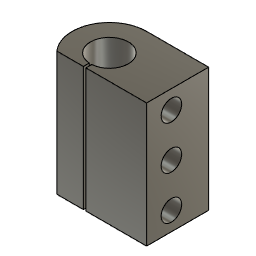
X-Idler (Autodesk Fusion 360 design; units mm, degrees)
Autodesk Fusion 360 part; units mm, degrees
note: some values were not read from the file. Set by a fixed rule: which sketch regions a step uses.
sketch "Skizze1" plane through (0, 0, 0) normal (0, 0, 1) x (1, 0, 0)
  circle A0 centre (0, 0) radius 7.65
  line L0 (15, -10) -> (-15, -10)
  line L1 (-15, -10) -> (-15, 15)
  line L2 (-15, 15) -> (15, 15)
  line L3 (15, 15) -> (15, -10)
  line L4 (0, 0) -> (0, -10)
  line L5 (0, -10) -> (-0.5, -10)
  line L6 (-0.5, -10) -> (0.5, -10)
  line L7 (0.5, -10) -> (0.5, -7.3)
  line L8 (0.5, -7.3) -> (-0.5, -7.3)
  line L9 (-0.5, -7.3) -> (-0.5, -10)
  circle A1 centre (0, 0) radius 15
  dimension "d1" = 15.3
  dimension "d4" = 15
  dimension "d5" = 10
  dimension "d6" = 15
  dimension "d7" = 25
  constraint coincident A0.centre L4.start
  constraint horizontal L0
  constraint vertical L1
  constraint horizontal L2
  constraint vertical L3
  constraint coincident L0 L4.end
  constraint perpendicular L0 L4
  constraint coincident L0 L5.end
  constraint horizontal L6
  constraint vertical L7
  constraint horizontal L8
  constraint vertical L9
  constraint concentric A0 A1
  constraint tangent L1 A1
  measures "d1" diameter of A0
  measures "d4" distance of A0.centre L3
  measures "d5" distance of A0.centre L0
  measures "d6" distance of A0.centre L1
  measures "d7" distance of L0.start L2.end
extrude "Extrusion1" add sketch "Skizze1" along normal blind 50 contours A0 L0 L7 L9 A1 | L0 L3 A1 | L2 L3 A1
sketch "Skizze2" plane through (15, 0, 0) normal (1, 0, 0) x (0, 1, 0)
  line L0 (-10, 0) -> (15, 0)
  line L1 (15, 0) -> (15, 50)
  line L2 (15, 50) -> (-10, 50)
  line L3 (-10, 50) -> (-10, 0)
  line L4 (-10, 25) -> (15, 25)
  circle A0 centre (0, 25) radius 4.15
  line L5 (0, 25) -> (0, 42.5)
  line L6 (0, 25) -> (0, 7.5)
  circle A1 centre (0, 42.5) radius 4.15
  circle A2 centre (0, 7.5) radius 4.15
  dimension "d10" = 8.3
  dimension "d11" = 10
  dimension "d22" = 17.5
  dimension "d23" = 8.3
  dimension "d24" = 8.3
  dimension "d25" = 17.5
  constraint midpoint L3 L4.start
  constraint midpoint L1 L4.end
  constraint coincident L4 A0.centre
  constraint coincident A0.centre L5.start
  constraint perpendicular L4 L5
  constraint perpendicular L4 L6
  constraint coincident L5.end A1.centre
  constraint coincident L6.end A2.centre
  measures "d10" diameter of A0
  measures "d11" distance of L3 A0.centre
  measures "d22" distance of A0.centre L5.end
  measures "d23" diameter of A1
  measures "d24" diameter of A2
  measures "d25" distance of A0.centre L6.end
extrude "Extrusion2" cut sketch "Skizze2" against normal blind 6 contours L4 A0 L5 | L4 A0 L6 | L4 A0 L6 | L4 A0 L5 | A1 | A2
extrude "Extrusion4" add 1 faces at (15, 11.3833, 25) along direction (1, 0, 0) blind 10
sketch "Skizze3" plane through (0, 15, 0) normal (0, 1, 0) x (-1, 0, 0)
  line L0 (-25, 0) -> (0, 0)
  line L1 (0, 50) -> (-25, 50)
  line L2 (-25, 25) -> (-18, 25)
  line L3 (-18, 25) -> (-18, 20.25)
  line L4 (-18, 25) -> (-18, 29.75)
  circle A0 centre (-18, 29.75) radius 1.5
  circle A1 centre (-18, 20.25) radius 1.5
  line L5 (0, 0) -> (0, 50)
  line L6 (-25, 50) -> (-25, 0)
  dimension "d15" = 7
  dimension "d16" = 4.75
  dimension "d17" = 4.75
  dimension "d18" = 3
  dimension "d19" = 3
  constraint perpendicular L2 L3
  constraint perpendicular L2 L4
  constraint coincident L4.end A0.centre
  constraint coincident L3.end A1.centre
  constraint midpoint L2.start L6
  constraint perpendicular L2 L6
  measures "d15" distance of L2.start L2.end
  measures "d16" distance of L2.end L3.end
  measures "d17" distance of L2.end L4.end
  measures "d18" diameter of A0
  measures "d19" diameter of A1
extrude "Extrusion3" cut sketch "Skizze3" against normal blind 5 contours A0 | A1
